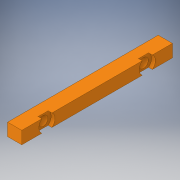
# Autodesk Inventor part: axil mount
Saved by Autodesk Inventor 2019 (Build 230136000, 136)
## iProperties
Created: 2019-03-12
Part Number: axil mount
Material: Generic
Document SubType Name: Modeling
Designer: Delta
Density: 1 g/cm^3
Appearance: Orange
Author: Delta
Autodesk Inventor part; units mm, degrees
ref_plane "YZ Plane" through (0, 0, 0) normal (1, 0, 0) x (0, 1, 0)
ref_plane "XZ Plane" through (0, 0, 0) normal (0, 1, 0) x (-1, 0, 0)
ref_plane "XY Plane" through (0, 0, 0) normal (0, 0, 1) x (1, 0, 0)
sketch "Sketch1" plane through (0, 0, 0) normal (0, 1, 0) x (-1, 0, 0)
  line L0 (0, 0) -> (14.351, 0)
  line L1 (14.351, 0) -> (14.351, -152.4)
  line L2 (14.351, -152.4) -> (0, -152.4)
  line L3 (0, -152.4) -> (0, 0)
  dimension "d0" = 152.4
  dimension "d1" = 14.351
  constraints: 8 end point, 2 parallel, 1 horizontal, 1 perpendicular
  measures "d0" distance of L0.end L1.end
  measures "d1" distance of L1.end L2.end
extrude "Extrusion1" add sketch "Sketch1" along normal blind 12.7
sketch "Sketch2" plane through (0, 0, 0) normal (1, 0, 0) x (0, 0, -1)
  circle A0 centre (25.4, 6.35) radius 4.7625
  circle A1 centre (127, 6.35) radius 4.7625
  line L0 (0, 12.7) -> (152.4, 12.7) projected
  line L1 (152.4, 0) -> (152.4, 12.7) projected
  point P0 (0, 0)
  dimension "d4" = 9.525
  dimension "d5" = 9.525
  dimension "d6" = 101.6
  dimension "d7" = 152.4
  dimension "d8" = 25.4
  dimension "d9" = 12.7
  dimension "d10" = 6.35
  dimension "d11" = 6.35
  constraints: 2 centre point
  measures "d4" diameter of A0
  measures "d5" diameter of A1
  measures "d6" distance of A0.centre A1.centre
  measures "d7" distance of L0.start L0.end
  measures "d8" distance from line of L1 A1.centre
  measures "d9" distance of L1.start L0.end
  measures "d10" distance from line of L0 A1.centre
  measures "d11" distance from line of L0 A0.centre
extrude "Extrusion2" cut sketch "Sketch2" against normal through all
sketch "Sketch4" plane through (0, 0, 0) normal (1, 0, 0) x (0, 0, -1)
  circle A0 centre (25.4, 6.35) radius 4.7625 projected
  circle A1 centre (127, 6.35) radius 4.7625 projected
  point P0 (0, 0)
  constraints: 2 coincident
hole "Hole1" at (0, 6.35, -25.4) at (0, 6.35, -127) direction (-1, 0, 0) diameter 16.256 depth 3.81
equation "\"d5\" = d4"
equation "\"d8\" = -0.5 * d6 + 0.5 * d7"
equation "\"d10\" = 0.5 * d9"
equation "\"d11\" = d10"
body "Solid1"
